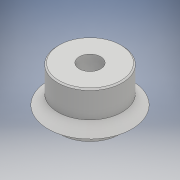
# Autodesk Inventor part: Engrenage_spiro_conique
Saved by Autodesk Inventor 2018 (Build 220112000, 112)
## iProperties
Created: 2019-11-06
Part Number: Engrenage_spiro_conique
Material: Generic
Document SubType Name: Modeling
Designer: hugo
Density: 1 g/cm^3
Appearance: Default
Author: hugo
Autodesk Inventor part; units mm, degrees
ref_plane "YZ Plane" through (0, 0, 0) normal (1, 0, 0) x (0, 1, 0)
ref_plane "XZ Plane" through (0, 0, 0) normal (0, 1, 0) x (-1, 0, 0)
ref_plane "XY Plane" through (0, 0, 0) normal (0, 0, 1) x (1, 0, 0)
sketch "Sketch1" plane through (0, 0, 0) normal (1, 0, 0) x (0, 1, 0)
  line L0 (0, 0) -> (12, 0)
  line L1 (12, 0) -> (12, -10)
  line L2 (12, -10) -> (15.63, -13.63)
  line L3 (15.63, -13.63) -> (11.1401, -17.61)
  line L4 (11.1401, -17.61) -> (9.515, -16)
  line L5 (9.515, -16) -> (0, -16)
  line L6 (0, -16) -> (0, 0)
  dimension "d0" = 12
  dimension "d1" = 10
  dimension "d2" = 15.63
  dimension "d3" = 13.63
  dimension "d4" = 17.61
  dimension "d5" = 6
  dimension "d6" = 9.515
  dimension "d7" = 16
  constraints: 14 end point, 2 horizontal, 2 perpendicular
  measures "d0" distance of L0.start L0.end
  measures "d1" distance of L0.end L1.end
  measures "d2" horizontal distance of L2.end L0.start
  measures "d3" vertical distance of L0.start L2.end
  measures "d4" vertical distance of L0.start L3.end
  measures "d5" distance of L2.end L3.end
  measures "d6" distance of L4.end L5.end
  measures "d7" distance between parallel lines of L0 L5
revolve "Revolution1" add sketch "Sketch1" angle 360 about axis through (0, 0, -16) along (0, 0, 1)
chamfer "Chamfer1" distance 0.5 angle 45 1 edges at (0, -12, 0)
sketch "Sketch2" plane through (0, 0, -16) normal (0, 0, -1) x (-1, 0, 0)
  circle A0 centre (0, 0) radius 4
  dimension "d12" = 8
  constraints: 1 centre point, 1 coincident
  measures "d12" diameter of A0
extrude "Extrusion1" cut sketch "Sketch2" against normal up to next
equation "\"d0\" = 0.5 * Be"
equation "\"d1\" = He"
equation "\"d2\" = 0.5 * De"
equation "\"d3\" = Ge"
equation "\"d4\" = Fe"
equation "\"d5\" = Je"
equation "\"d6\" = 0.5 * Ke"
equation "\"d7\" = Le"
equation "\"d12\" = Ae"
equation "\"Ae\" = 8"
equation "\"Be\" = 24"
equation "\"De\" = 31.26"
equation "\"Ee\" = 28"
equation "\"Fe\" = 17.61"
equation "\"Ge\" = 13.63"
equation "\"He\" = 10"
equation "\"Je\" = 6"
equation "\"Ke\" = 19.03"
equation "\"Le\" = 16"
body "Solid1"
